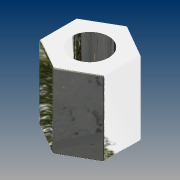
# Autodesk Inventor part: Nut
Saved by Autodesk Inventor 2015 (Build 190159000, 159)
## iProperties
Created: 2021-03-29
Part Number: Nut
Material: Iron, Malleable
Document SubType Name: Modeling
Designer: Diptanshu Das
Density: 7.1 g/cm^3
Appearance: Brindle
Author: Diptanshu Das
Autodesk Inventor part; units mm, degrees
ref_plane "YZ Plane" through (0, 0, 0) normal (1, 0, 0) x (0, 1, 0)
ref_plane "XZ Plane" through (0, 0, 0) normal (0, 1, 0) x (-1, 0, 0)
ref_plane "XY Plane" through (0, 0, 0) normal (0, 0, 1) x (1, 0, 0)
sketch "Sketch1" plane through (0, 0, 0) normal (0, 0, 1) x (1, 0, 0)
  circle A0 centre (0, 0) radius 50
  circle A1 centre (0, 0) radius 25
  dimension "d0" = 100
  dimension "d1" = 50
  constraints: 2 centre point, 2 coincident
  measures "d0" diameter of A0
  measures "d1" diameter of A1
extrude "Extrusion1" add sketch "Sketch1" along normal blind 100
sketch "Sketch2" plane through (0, 0, 100) normal (0, 0, 1) x (1, 0, 0)
  circle A0 centre (0, 0) radius 50 projected
  line L0 (0, 50) -> (43.3013, 25)
  line L1 (43.3013, 25) -> (43.3013, -25)
  line L2 (43.3013, -25) -> (0, -50)
  line L3 (0, -50) -> (-43.3013, -25)
  line L4 (-43.3013, -25) -> (-43.3013, 25)
  line L5 (-43.3013, 25) -> (0, 50)
  circle A1 centre (0, 0) radius 50
  dimension "d4" = 0
  constraints: 12 end point, 1 centre point, 1 coincident, 1 vertical alignment, 14 other
extrude "Extrusion2" cut sketch "Sketch2" against normal blind 100 contours A0 L1 | L0 A0 | A0 L2 | L5 A0 | A0 L3 | L4 A0
fillet "Fillet1" radius 2 12 edges at (0, 50, 50) (21.6506, 37.5, 100) (-21.6506, 37.5, 100) (43.3013, 25, 50) (43.3013, -25, 50) (43.3013, 0, 100) (-43.3013, 25, 50) (-43.3013, 0, 100) (-43.3013, -25, 50) (-21.6506, -37.5, 100) (0, -50, 50) (21.6506, -37.5, 100)
fillet "Fillet2" radius 2 12 edges at (0, 49.6906, 0) (21.6506, 37.5, 0) (43.0333, 24.8453, 0) (43.3013, 0, 0) (43.0333, -24.8453, 0) (21.6506, -37.5, 0) (0, -49.6906, 0) (-21.6506, -37.5, 0) (-43.0333, -24.8453, 0) (-43.3013, 0, 0) (-43.0333, 24.8453, 0) (-21.6506, 37.5, 0)
body "Solid1"
